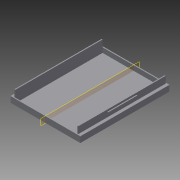
# Autodesk Inventor part: top2
Saved by Autodesk Inventor 2015 SP2 (Build 190223200, 223)
## iProperties
Created: 2016-03-10
Part Number: top2
Material: Generic
Document SubType Name: Modeling
Designer: mca20
Density: 1 g/cm^3
Appearance: Default
Author: mca20
Autodesk Inventor part; units mm, degrees
ref_plane "YZ Plane" through (0, 0, 0) normal (1, 0, 0) x (0, 1, 0)
ref_plane "XZ Plane" through (0, 0, 0) normal (0, 1, 0) x (-1, 0, 0)
ref_plane "XY Plane" through (0, 0, 0) normal (0, 0, 1) x (1, 0, 0)
sketch "Sketch1" plane through (0, 0, 0) normal (0, 1, 0) x (-1, 0, 0)
  line L0 (0, 0) -> (69, 0)
  line L1 (69, 0) -> (69, -92)
  line L2 (69, -92) -> (0, -92)
  line L3 (0, -92) -> (0, 0)
  dimension "d0" = 69
  dimension "d1" = 92
  constraints: 8 end point, 2 parallel, 1 horizontal, 1 perpendicular
  measures "d0" distance of L1.end L2.end
  measures "d1" distance of L0.end L1.end
extrude "Extrusion1" add sketch "Sketch1" along normal blind 1
sketch "Sketch2" plane through (0, 1, 0) normal (0, 1, 0) x (1, 0, 0)
  line L0 (-69, 0) -> (0, 0) projected
  line L1 (0, 0) -> (0, 92) projected
  line L2 (0, 92) -> (-69, 92) projected
  line L3 (-69, 92) -> (-69, 0) projected
  line L4 (-68, 1) -> (-1, 1)
  line L5 (-1, 1) -> (-1, 91)
  line L6 (-1, 91) -> (-68, 91)
  line L7 (-68, 91) -> (-68, 1)
  line L8 (-67.5, 1) -> (-67.5, 91)
  line L9 (-1.5, 1) -> (-1.5, 91)
  dimension "d4" = 1
  dimension "d5" = 0.5
  dimension "d6" = 0.5
  constraints: 12 end point, 4 point on line, 2 perpendicular, 3 other
  measures "d4" distance between parallel lines of L3 L7
  measures "d5" distance between parallel lines of L8 L7
  measures "d6" distance between parallel lines of L5 L9
extrude "Extrusion2" add sketch "Sketch2" along normal blind 5 contours L3 L2 L1 L0 | L7 L6 L8 L4 | L9 L6 L5 L4
sketch "Sketch3" plane through (0, 1, 0) normal (0, 1, 0) x (1, 0, 0)
  line L0 (-67.5, 91) -> (-67.5, 1) projected
  line L1 (-67.5, 1) -> (-1.5, 1) projected
  line L2 (-1.5, 1) -> (-1.5, 91) projected
  line L3 (-1.5, 91) -> (-67.5, 91) projected
  line L4 (-67.5, 1) -> (-1.5, 1) projected
  line L5 (-66.5, 1) -> (-66.5, 91)
  line L6 (-2.5, 1) -> (-2.5, 91)
  point P0 (0, 0)
  dimension "d9" = 1
  dimension "d10" = 1
  constraints: 4 end point, 4 point on line, 2 perpendicular
  measures "d9" distance between parallel lines of L0 L5
  measures "d10" distance between parallel lines of L2 L6
extrude "Extrusion3" add sketch "Sketch3" along normal blind 12 contours L3 L5 L1 L0 | L3 L2 L1 L6
sketch "Sketch4" plane through (-1.5, 6, -91) normal (1, 0, 0) x (0, 0, -1)
  line L0 (-90, 0) -> (-90, 7) projected
  line L1 (-90, 4) -> (-90, 5)
  line L2 (0, 0) -> (0, 7) projected
  line L3 (-90, 7) -> (0, 7) projected
  line L4 (-60, 5) -> (-30, 5)
  line L5 (-30, 5) -> (-30, 4)
  line L6 (-30, 4) -> (-60, 4)
  line L7 (-60, 4) -> (-60, 5)
  line L8 (0, 0) -> (-90, 0) projected
  point P0 (-91, -6)
  dimension "d21" = 1
  dimension "d22" = 2
  dimension "d23" = 4
  dimension "d24" = 30
  dimension "d25" = 30
  constraints: 10 end point, 2 parallel, 1 horizontal, 1 perpendicular, 1 point on line
  measures "d21" distance between parallel lines of L6 L4
  measures "d22" distance between parallel lines of L4 L3
  measures "d23" distance between parallel lines of L8 L6
  measures "d24" distance between parallel lines of L0 L7
  measures "d25" distance between parallel lines of L2 L5
ref_plane "Work Plane1" through (-34.5, 0, 0) normal (1, 0, 0) x (0, 0, -1)
extrude "Extrusion5" add sketch "Sketch4" along normal blind 1 contours L4 L5 L6 L7
mirror "Mirror2" about plane through (-34.5, 0, 0) normal (1, 0, 0) of "Extrusion5"
sketch "Sketch5" plane through (0, 0, 0) normal (1, 0, 0) x (0, 0, -1)
  line L0 (92, 0) -> (0, 0) projected
  line L1 (92, 0) -> (92, 6) projected
  line L2 (0, 6) -> (92, 6) projected
  line L3 (0, 0) -> (0, 6) projected
extrude "Extrusion6" add sketch "Sketch5" along normal blind 1.5
sketch "Sketch6" plane through (-69, 0, -92) normal (-1, 0, 0) x (0, 0, 1)
  line L0 (92, 0) -> (0, 0) projected
  line L1 (92, 0) -> (92, 6) projected
  line L2 (0, 6) -> (92, 6) projected
  line L3 (0, 0) -> (0, 6) projected
extrude "Extrusion7" add sketch "Sketch6" along normal blind 1.5
body "Solid1"
